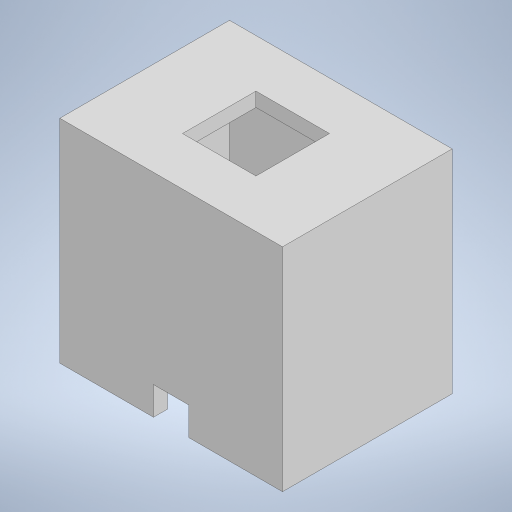
# Autodesk Inventor part: button_holder
Saved by Autodesk Inventor 2023 (Build 270158000, 158)
## iProperties
Created: 2023-10-25
Part Number: button_holder
Material: Generic
Document SubType Name: Modeling
Designer: zskus
Density: 1 g/cm^3
Appearance: Default
Author: zskus
Autodesk Inventor part; units mm, degrees
ref_plane "YZ Plane" through (0, 0, 0) normal (1, 0, 0) x (0, 1, 0)
ref_plane "XZ Plane" through (0, 0, 0) normal (0, 1, 0) x (-1, 0, 0)
ref_plane "XY Plane" through (0, 0, 0) normal (0, 0, 1) x (1, 0, 0)
sketch "Sketch1" plane through (0, 0, 0) normal (0, 1, 0) x (-1, 0, 0)
  line L0 (8.7312, 6.35) -> (-8.7313, 6.35)
  line L1 (-8.7313, 6.35) -> (-8.7312, -6.35)
  line L2 (-8.7312, -6.35) -> (8.7313, -6.35)
  line L3 (8.7313, -6.35) -> (8.7312, 6.35)
  line L4 (3.302, -3.302) -> (-3.302, -3.302)
  line L5 (-3.302, -3.302) -> (-3.302, 3.302)
  line L6 (-3.302, 3.302) -> (3.302, 3.302)
  line L7 (3.302, 3.302) -> (3.302, -3.302)
  point P0 (0, 0)
  dimension "d0" = 12.7
  dimension "d1" = 17.4625
  dimension "d2" = 6.35
  dimension "d3" = 8.7312
  dimension "d16" = 6.604
  dimension "d17" = 6.604
  dimension "d18" = 3.302
  dimension "d19" = 3.302
  constraints: 16 end point, 4 parallel, 2 horizontal, 2 perpendicular
  measures "d0" distance of L2.end L0.start
  measures "d1" distance of L0.start L0.end
  measures "d2" distance from line of L0 point (0, 0)
  measures "d3" distance from line of L1 point (0, 0)
  measures "d16" distance of L4.start L4.end
  measures "d17" distance of L4.end L5.end
  measures "d18" horizontal distance of point (0, 0) L4.end
  measures "d19" horizontal distance of point (0, 0) L4.start
extrude "Extrusion1" add sketch "Sketch1" along normal blind 1.27
sketch "Sketch2" plane through (0, 1.27, 0) normal (0, 1, 0) x (1, 0, 0)
  line L0 (8.7313, -6.35) -> (8.7312, 6.35) projected
  line L1 (8.7312, 6.35) -> (-8.7313, 6.35) projected
  line L2 (-8.7313, 6.35) -> (-8.7312, -6.35) projected
  line L3 (-8.7312, -6.35) -> (8.7313, -6.35) projected
  line L4 (-10.0012, -7.62) -> (-10.0013, 7.62)
  line L5 (-10.0013, 7.62) -> (10.0013, 7.62)
  line L6 (10.0013, 7.62) -> (10.0013, -7.62)
  line L7 (10.0013, -7.62) -> (-10.0012, -7.62)
  point P0 (0, 0)
  dimension "d7" = 1.27
  constraints: 8 end point, 3 other
  measures "d7" distance between parallel lines of L2 L4
extrude "Extrusion2" add sketch "Sketch2" against normal blind 19.05
sketch "Sketch3" plane through (-10.0012, 1.27, 7.62) normal (0, 0, 1) x (1, 0, 0)
  line L0 (0, 0) -> (20.0025, 0) projected
  line L1 (0, 0) -> (0, -19.05) projected
  line L2 (20.0025, -19.05) -> (0, -19.05) projected
  line L3 (20.0025, 0) -> (20.0025, -19.05) projected
  line L4 (0, -19.05) -> (20.0025, -19.05) projected
  line L5 (8.4138, -19.05) -> (11.5888, -19.05)
  line L6 (11.5888, -19.05) -> (11.5887, -16.51)
  line L7 (11.5887, -16.51) -> (8.4138, -16.51)
  line L8 (8.4138, -16.51) -> (8.4138, -19.05)
  point P0 (10.0012, -1.27)
  point P1 (10.0012, -16.51)
  dimension "d10" = 3.175
  dimension "d11" = 20.0025
  dimension "d12" = 10.0013
  dimension "d13" = 2.54
  constraints: 8 end point, 2 parallel, 1 horizontal, 1 midpoint, 1 perpendicular, 1 point on line
  measures "d10" distance of L6.end L7.end
  measures "d11" distance of L0.start L0.end
  measures "d12" distance from line of L3 point (10.001, -16.51)
  measures "d13" distance of L5.end L6.end
extrude "Extrusion3" cut sketch "Sketch3" against normal blind 3.81 contours L8 L7 L6 L2
equation "\"d2\" = 0.5 * d0"
equation "\"d3\" = 0.5 * d1"
equation "\"d18\" = 0.5 * d16"
equation "\"d19\" = 0.5 * d17"
equation "\"d12\" = 0.5 * d11"
body "Solid1"
